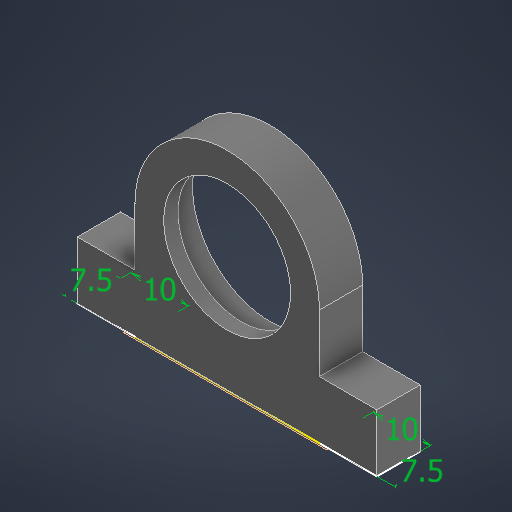
# Autodesk Inventor part: Adafruit_1528_4699_ND_House_02
Saved by Autodesk Inventor 2026.2 (Build 302298000, 298)
## iProperties
Created: 2026-02-02
Part Number: Adafruit_1528_4699_ND_House_02
Material: Generic
Document SubType Name: Modeling
Designer: vckot
Density: 1 g/cm^3
Appearance: Gray
Author: vckot
Autodesk Inventor part; units mm, degrees
ref_plane "YZ Plane" through (0, 0, 0) normal (1, 0, 0) x (0, 1, 0)
ref_plane "XY Plane" through (0, 0, 0) normal (0, 0, 1) x (1, 0, 0)
sketch "Sketch1" plane through (0, 0, 0) normal (0, 0, 1) x (1, 0, 0)
  circle A0 centre (0, 0) radius 13.5
  circle A1 centre (0, 0) radius 16
  circle A2 centre (0, 0) radius 11
  dimension "d0" = 27
  dimension "d1" = 32
  dimension "d2" = 22
  constraints: 3 centre point, 3 coincident
  measures "d0" diameter of A0
  measures "d1" diameter of A1
  measures "d2" diameter of A2
extrude "Extrusion1" add sketch "Sketch1" along normal blind 2.5 contours A0 | A1
extrude "Extrusion2" add sketch "Sketch1" against normal blind 5 contours A1
ref_plane "Work Plane1" through (0, -20, 0) normal (0, 1, 0) x (-1, 0, 0)
sketch "Sketch2" plane through (0, -20, 0) normal (0, 1, 0) x (-1, 0, 0)
  line L0 (-16, -5) -> (16, -5) projected
  line L1 (16, 2.5) -> (-16, 2.5) projected
  line L2 (16, -5) -> (16, 2.5) projected
  line L3 (-16, -5) -> (-16, 2.5) projected
  line L4 (-16, 2.5) -> (-26, 2.5)
  line L5 (-26, 2.5) -> (-26, -5)
  line L6 (-26, -5) -> (-16, -5)
  line L7 (-16, -5) -> (-16, 2.5)
  line L8 (16, 2.5) -> (26, 2.5)
  line L9 (26, 2.5) -> (26, -5)
  line L10 (26, -5) -> (16, -5)
  line L11 (16, -5) -> (16, 2.5)
  point P0 (0, 0)
  dimension "d8" = 10
  dimension "d9" = 7.5
  dimension "d10" = 10
  dimension "d11" = 7.5
  constraints: 16 end point, 4 parallel, 2 horizontal, 2 perpendicular
  measures "d8" distance of L6.end L5.end
  measures "d9" distance of L4.end L5.end
  measures "d10" distance of L9.end L10.end
  measures "d11" distance of L8.end L9.end
extrude "Extrusion3" add sketch "Sketch2" along normal blind 20 contours L3 L1 L2 L0
delete faces "Delete Face1" heal yes whole lump no faces at (-3.6667, 0, -3.3333)
extrude "Extrusion4" add sketch "Sketch2" along normal blind 10 contours L6 L5 L4 L3 | L2 L8 L9 L10
body "Solid1"
